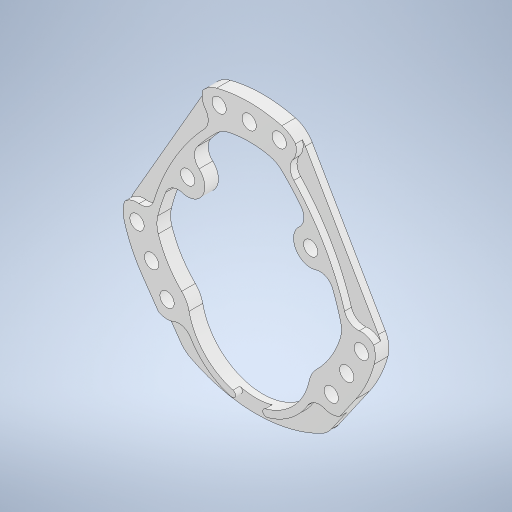
# Autodesk Inventor part: Support Ring
Saved by Autodesk Inventor 2023.2 (Build 272271000, 271)
## iProperties
Created: 2023-06-11
Part Number: Support Ring
Material: UHMW, White
Document SubType Name: Modeling
Designer: Nathan Cai
Mass: 20.1005 g
Surface Area: 140.616 cm^2
Volume: 21.3835 cm^3
Density: 0.94 g/cm^3
Appearance: Smooth - White
Author: Nathan Cai
Autodesk Inventor part; units mm, degrees
ref_plane "YZ Plane" through (0, 0, 0) normal (1, 0, 0) x (0, 1, 0)
ref_plane "XZ Plane" through (0, 0, 0) normal (0, 1, 0) x (-1, 0, 0)
ref_plane "XY Plane" through (0, 0, 0) normal (0, 0, 1) x (1, 0, 0)
sketch "Sketch1" plane through (0, 0, 0) normal (0, 0, 1) x (1, 0, 0)
  circle A0 centre (0, 0) radius 60.325
  line L0 (0, 0) -> (0, 60.325) construction
  circle A1 centre (0, 52.3875) radius 7.9375 construction
  circle A2 centre (0, 52.3875) radius 3.302
  circle A3 centre (-45.3689, -26.1937) radius 3.302
  circle A4 centre (45.3689, -26.1938) radius 3.302
  circle A5 centre (0, 0) radius 44.45
  circle A6 centre (0, -31.75) radius 28.575 construction
  circle A7 centre (0, -31.75) radius 28.575
  circle A8 centre (0, 0) radius 66.675
  line L1 (0, 0) -> (-33.3375, -57.7422)
  line L2 (0, 0) -> (33.3375, -57.7422)
  line L3 (-33.3375, -57.7422) -> (-49.5411, -34.4207)
  line L4 (33.3375, -57.7422) -> (49.5411, -34.4207)
  circle A9 centre (-45.3689, -26.1937) radius 7.9375 construction
  circle A10 centre (45.3689, -26.1938) radius 7.9375 construction
  circle A11 centre (0, 52.3875) radius 4.7625 construction
  circle A12 centre (-45.3689, -26.1937) radius 4.7625 construction
  circle A13 centre (45.3689, -26.1938) radius 4.7625 construction
  circle A14 centre (28.575, 15.9015) radius 26.9875
  circle A15 centre (28.575, 15.9015) radius 3.302
  circle A16 centre (28.575, 15.9015) radius 7.9375
  circle A17 centre (-28.575, 15.9015) radius 3.302
  circle A18 centre (-28.575, 15.9015) radius 7.9375
  point P0 (-28.4756, -34.1313)
  point P1 (28.4756, -34.1313)
  point P2 (33.3375, -57.7422)
  point P3 (49.5411, -34.4207)
  dimension "d12" = 133.35
  dimension "d0" = 120.65
  dimension "d1" = 15.875
  dimension "d2" = 6.604
  dimension "d5" = 360
  dimension "d7" = 88.9
  dimension "d10" = 57.15
  dimension "d11" = 57.15
  dimension "d13" = 30
  dimension "d17" = 360
  dimension "d21" = 9.525
  dimension "d24" = 360
  dimension "d61" = 53.975
  dimension "d62" = 28.575
  dimension "d63" = 6.604
  dimension "d64" = 15.875
  constraints: 18 centre point, 10 end point, 9 coincident, 4 symmetric about line, 4 tangent, 2 point on circle, 2 point on line, 1 vertical, 26 other
  measures "d0" diameter of A0
  measures "d1" diameter of A1
  measures "d2" diameter of A2
  measures "d7" diameter of A5
  measures "d10" diameter of A6
  measures "d11" diameter of A7
  measures "d13" angle of L0 L1
  measures "d21" diameter of A11
  measures "d61" diameter of A14
  measures "d62" distance from line of L0 A14.centre
  measures "d63" diameter of A15
  measures "d64" diameter of A16
extrude "Extrusion1" add sketch "Sketch1" along normal blind 6.35 contours A0 L2 A7 A5 A14 L1 | A0 L1 L3 | L4 L2 A0 | L1 A7 A0 | A0 L2 A8 L1 | A0 A7 L2 | A14 A5 | A16 | A18 picked at (43.5815, 23.2371)
fillet "Fillet1" radius 12.7 4 edges at (-28.4756, -34.1313, 3.175) (28.4756, -34.1312, 3.175) (33.3375, -57.7422, 3.175) (-33.3375, -57.7422, 3.175)
sketch "Sketch2" plane through (0, 0, 0) normal (0, 0, -1) x (-1, 0, 0)
  point P0 (-38.1661, -38.1661)
  point P1 (-52.1358, -13.9698)
  point P2 (-13.9698, 52.1358)
  point P3 (13.9698, 52.1358)
  point P4 (52.1358, -13.9698)
  point P5 (38.1661, -38.1661)
hole "Hole1" at (38.1661, -38.1661, 0) at (52.1358, -13.9698, 0) at (13.9698, 52.1358, 0) at (-13.9698, 52.1358, 0) at (-52.1358, -13.9698, 0) at (-38.1661, -38.1661, 0) direction (0, 0, 1) diameter 6.604 end through all
sketch "Sketch3" plane through (0, 0, 0) normal (0, 0, -1) x (-1, 0, 0)
  circle A0 centre (13.9698, 52.1358) radius 3.302 projected
  circle A1 centre (13.9698, 52.1358) radius 7.9375
  circle A2 centre (-13.9698, 52.1358) radius 3.302 projected
  circle A3 centre (-13.9698, 52.1358) radius 7.9375
  circle A4 centre (-52.1358, -13.9698) radius 7.9375
  circle A5 centre (-38.1661, -38.1661) radius 7.9375
  circle A6 centre (38.1661, -38.1661) radius 7.9375
  circle A7 centre (52.1358, -13.9698) radius 7.9375
  line L0 (20.8438, 56.1046) -> (59.0099, -10.001)
  line L1 (-59.0099, -10.001) -> (-20.8438, 56.1046)
  line L2 (38.1661, -46.1036) -> (-38.1661, -46.1036)
  arc A8 (44.3097, -15.2947) -> (8.9093, 46.0207) centre (-55.8649, -32.2536) ccw
  arc A9 (-8.9093, 46.0207) -> (-44.3097, -15.2947) centre (55.8649, -32.2536) ccw
  arc A10 (-35.4004, -30.726) -> (35.4004, -30.726) centre (0, 64.5072) ccw
  circle A11 centre (0, 0) radius 61.9125
  circle A12 centre (0, 52.3875) radius 3.302 projected
  circle A13 centre (0, 52.3875) radius 7.9375
  point P0 (-44.3097, -15.2947)
  point P1 (-8.9093, 46.0207)
  point P2 (-16.0241, 59.8029)
  point P3 (-59.8029, -16.0241)
  point P4 (59.8029, -16.0241)
  point P5 (16.0241, 59.8029)
  dimension "d33" = 15.875
  dimension "d34" = 15.875
  dimension "d37" = 360
  dimension "d41" = 360
  dimension "d43" = 101.6
  dimension "d46" = 360
  dimension "d50" = 15.875
  constraints: 11 centre point, 10 point on circle, 6 end point, 5 tangent, 4 coincident, 36 other
  measures "d33" diameter of A1
  measures "d34" diameter of A3
  measures "d43" radius of A8
  measures "d50" diameter of A13
extrude "Extrusion2" add sketch "Sketch3" against normal blind 6.35 contours A1 L0 A7 A8 | A3 A9 A4 L1
extrude "Extrusion3" cut sketch "Sketch3" against normal through all contours A1 A11 A7 L0 | A3 L1 A4 A11
fillet "Fillet3" radius 12.7 8 edges at (-20.4179, 56.7645, 3.175) (20.4179, 56.7645, 3.175) (12.9034, 42.5359, 3.175) (-12.9034, 42.5359, 3.175) (-43.2889, -10.0933, 3.175) (43.2889, -10.0933, 3.175) (59.3685, -10.6998, 3.175) (-59.3685, -10.6998, 3.175)
sketch "Sketch4" plane through (0, 0, 6.35) normal (0, 0, 1) x (1, 0, 0)
  arc A0 (-56.9, -6.3464) -> (-58.1418, -16.0821) centre (-45.9014, -12.6964) ccw projected
  arc A1 (-58.1418, -16.0821) -> (-49.5411, -34.4207) centre (0, 0) ccw projected
  line L0 (-49.5411, -34.4207) -> (-35.0482, -55.2801) projected
  arc A2 (-35.0482, -55.2801) -> (-30.411, -59.3357) centre (-24.6185, -48.0337) ccw projected
  arc A3 (-30.411, -59.3357) -> (30.411, -59.3357) centre (0, 0) ccw projected
  arc A4 (30.411, -59.3357) -> (35.0482, -55.2801) centre (24.6185, -48.0337) ccw projected
  line L1 (35.0482, -55.2801) -> (49.5411, -34.4207) projected
  arc A5 (49.5411, -34.4207) -> (58.1418, -16.0821) centre (0, 0) ccw projected
  arc A6 (58.1418, -16.0821) -> (56.9, -6.3464) centre (45.9014, -12.6964) ccw projected
  line L2 (56.9, -6.3464) -> (22.9538, 52.45) projected
  arc A7 (22.9538, 52.45) -> (15.1434, 58.3934) centre (11.9553, 46.1) ccw projected
  arc A8 (15.1434, 58.3934) -> (-15.1434, 58.3934) centre (0, 0) ccw projected
  arc A9 (-15.1434, 58.3934) -> (-22.9538, 52.45) centre (-11.9553, 46.1) ccw projected
  line L3 (-22.9538, 52.45) -> (-56.9, -6.3464) projected
  arc A10 (31.3763, -31.4854) -> (42.2431, -13.832) centre (0, 0) ccw projected
  arc A11 (31.3763, -31.4854) -> (27.9283, -37.7947) centre (40.3409, -40.4813) ccw projected
  arc A12 (-27.9283, -37.7947) -> (27.9283, -37.7947) centre (0, -31.75) ccw projected
  arc A13 (-27.9283, -37.7947) -> (-31.3763, -31.4854) centre (-40.3409, -40.4813) ccw projected
  arc A14 (-42.2431, -13.832) -> (-31.3763, -31.4854) centre (0, 0) ccw projected
  arc A15 (-42.4649, -6.6838) -> (-42.2431, -13.832) centre (-30.1736, -9.88) ccw projected
  arc A16 (-35.5427, 12.0995) -> (-42.4649, -6.6838) centre (55.8649, -32.2536) ccw projected
  arc A17 (-9.1427, 43.4996) -> (-15.4441, 40.1175) centre (-6.5305, 31.0711) ccw projected
  arc A18 (9.1427, 43.4996) -> (-9.1427, 43.4996) centre (0, 0) ccw projected
  arc A19 (15.4441, 40.1175) -> (9.1427, 43.4996) centre (6.5305, 31.0711) ccw projected
  arc A20 (28.8506, 23.8342) -> (15.4441, 40.1175) centre (-55.8649, -32.2536) ccw projected
  arc A21 (42.2431, -13.832) -> (42.4649, -6.6838) centre (30.1736, -9.88) ccw projected
  circle A22 centre (-52.1358, -13.9698) radius 3.302 projected
  circle A23 centre (13.9698, 52.1358) radius 3.302 projected
  circle A24 centre (38.1661, -38.1661) radius 3.302 projected
  circle A25 centre (52.1358, -13.9698) radius 3.302 projected
  circle A26 centre (-13.9698, 52.1358) radius 3.302 projected
  circle A27 centre (-38.1661, -38.1661) radius 3.302 projected
  circle A28 centre (0, 52.3875) radius 3.302 projected
  circle A29 centre (-45.3689, -26.1937) radius 3.302 projected
  circle A30 centre (45.3689, -26.1938) radius 3.302 projected
  arc A31 (17.6725, 42.3791) -> (9.7957, 46.6067) centre (6.5305, 31.0711) ccw
  arc A32 (9.7957, 46.6067) -> (-9.7957, 46.6067) centre (0, 0) ccw
  arc A33 (-9.7957, 46.6067) -> (-17.6725, 42.3791) centre (-6.5305, 31.0711) ccw
  arc A34 (-17.6725, 42.3791) -> (-45.5377, -5.8847) centre (55.8649, -32.2536) ccw
  arc A35 (-45.5377, -5.8847) -> (-45.2604, -14.82) centre (-30.1736, -9.88) ccw
  arc A36 (-45.2604, -14.82) -> (-33.6174, -33.7344) centre (0, 0) ccw
  arc A37 (-31.0315, -38.4663) -> (-33.6174, -33.7344) centre (-40.3409, -40.4813) ccw
  arc A38 (-31.0315, -38.4663) -> (31.0315, -38.4663) centre (0, -31.75) ccw
  arc A39 (33.6174, -33.7344) -> (31.0315, -38.4663) centre (40.3409, -40.4813) ccw
  arc A40 (33.6174, -33.7344) -> (45.2604, -14.82) centre (0, 0) ccw
  arc A41 (45.2604, -14.82) -> (45.5377, -5.8847) centre (30.1736, -9.88) ccw
  arc A42 (45.5377, -5.8847) -> (17.6725, 42.3791) centre (-55.8649, -32.2536) ccw
  circle A43 centre (52.1358, -13.9698) radius 7.9375
  circle A44 centre (38.1661, -38.1661) radius 7.9375
  line L4 (0, 0) -> (0, -60.325) construction
  arc A45 (-27.9283, -37.7947) -> (27.9283, -37.7947) centre (0, -31.75) ccw projected
  circle A46 centre (13.9698, 52.1358) radius 3.302 projected
  circle A47 centre (13.9698, 52.1358) radius 7.9375
  circle A48 centre (-52.1358, -13.9698) radius 7.9375
  circle A49 centre (-38.1661, -38.1661) radius 7.9375
  circle A50 centre (-13.9698, 52.1358) radius 7.9375
  arc A51 (28.8506, 23.8342) -> (35.5427, 12.0995) centre (28.575, 15.9015) ccw projected
  arc A52 (42.4649, -6.6838) -> (35.5427, 12.0995) centre (-55.8649, -32.2536) ccw projected
  arc A53 (-35.5427, 12.0995) -> (-28.8506, 23.8342) centre (-28.575, 15.9015) ccw projected
  arc A54 (-15.4441, 40.1175) -> (-28.8506, 23.8342) centre (55.8649, -32.2536) ccw projected
  point P0 (-57.8882, -8.5004)
  point P1 (-46.019, -8.9112)
  point P2 (-15.2922, 44.3093)
  point P3 (-21.5826, 54.3829)
  point P4 (21.5826, 54.3829)
  point P5 (15.2922, 44.3093)
  point P6 (46.019, -8.9112)
  point P7 (57.8882, -8.5004)
  point P8 (42.1818, -45.0129)
  point P9 (30.5492, -40.3992)
  point P10 (-30.5492, -40.3992)
  point P11 (-42.1818, -45.0129)
  dimension "d54" = 3.175
  dimension "d55" = 15.875
  dimension "d56" = 15.875
  dimension "d57" = 15.875
  constraints: 26 point on circle, 18 centre point, 3 coincident, 3 symmetric about line, 2 end point, 14 other
  measures "d54" radial gap between concentric circles of A20 A42
  measures "d55" diameter of A43
  measures "d56" diameter of A44
  measures "d57" diameter of A47
extrude "Extrusion4" cut sketch "Sketch4" against normal blind 3.175 contours L3 A9 A50 A33 A34 A35 A48 A0 | A49 A38 A44 L1 A4 A3 A2 L0 | A7 L2 A6 A43 A41 A42 A31 A47
fillet "Fillet4" radius 6.35 10 edges at (46.019, -8.9112, 4.7625) (15.2922, 44.3093, 4.7625) (-15.2922, 44.3093, 4.7625) (-46.019, -8.9112, 4.7625) (-30.5492, -40.3992, 4.7625) (30.5492, -40.3992, 4.7625) (35.5427, 12.0995, 3.175) (28.8506, 23.8342, 3.175) (-35.5427, 12.0995, 3.175) (-28.8506, 23.8342, 3.175)
sketch "Sketch5" plane through (0, 0, 6.35) normal (0, 0, 1) x (1, 0, 0)
  arc A0 (-27.9283, -37.7947) -> (27.9283, -37.7947) centre (0, -31.75) ccw projected
  line L0 (0, 0) -> (0, -31.75) construction
  circle A1 centre (0, -60.325) radius 6.35
  dimension "d65" = 12.7
  constraints: 2 end point, 1 centre point, 1 point on circle, 1 vertical
  measures "d65" diameter of A1
extrude "Extrusion5" cut sketch "Sketch5" against normal up to surface (3.175 mm away)
fillet "Fillet5" radius 1.5875 4 edges at (-5.7725, -62.9708, 4.7625) (5.7725, -62.9708, 4.7625) (6.3107, -59.6194, 4.7625) (-6.3107, -59.6194, 4.7625)
body "Solid1"
